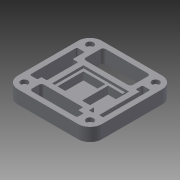
# Autodesk Inventor part: 16 pin holder
Saved by Autodesk Inventor 2015 (Build 190159000, 159)
## iProperties
Created: 2014-12-11
Part Number: 16 pin holder
Material: Generic
Document SubType Name: Modeling
Designer: Purple
Density: 1 g/cm^3
Appearance: Default
Author: Purple
Autodesk Inventor part; units mm, degrees
ref_plane "YZ Plane" through (0, 0, 0) normal (1, 0, 0) x (0, 1, 0)
ref_plane "XZ Plane" through (0, 0, 0) normal (0, 1, 0) x (-1, 0, 0)
sketch "Sketch1" plane through (0, 0, 0) normal (0, 1, 0) x (-1, 0, 0)
  line L0 (30, 30) -> (-30, 30)
  line L1 (-30, 30) -> (-30, -30)
  line L2 (-30, -30) -> (30, -30)
  line L3 (30, -30) -> (30, 30)
  line L4 (30, 30) -> (-30, -30) construction
  line L5 (-30, 30) -> (30, -30) construction
  point P0 (0, 0)
  dimension "d0" = 60
  dimension "d1" = 60
  constraints: 12 end point, 2 midpoint, 2 parallel, 1 horizontal, 1 perpendicular
  measures "d0" distance of L2.end L1.end
  measures "d1" distance of L0.end L1.end
extrude "Extrusion1" add sketch "Sketch1" along normal blind 10
fillet "Fillet1" radius 7 4 edges at (30, 5, 30) (30, 5, -30) (-30, 5, 30) (-30, 5, -30)
sketch "Sketch2" plane through (0, 10, 0) normal (0, 1, 0) x (1, 0, 0)
  line L0 (-30, 30) -> (30, 30)
  line L1 (30, 30) -> (30, -30)
  line L2 (30, -30) -> (-30, -30)
  line L3 (-30, -30) -> (-30, 30)
  line L4 (-30, 30) -> (30, -30) construction
  line L5 (30, 30) -> (-30, -30) construction
  line L6 (25, -25) -> (25, 25)
  line L7 (25, 25) -> (-25, 25)
  line L8 (-25, 25) -> (-25, -25)
  line L9 (-25, -25) -> (25, -25)
  circle A0 centre (25, -25) radius 2.75
  circle A1 centre (-25, -25) radius 2.75
  circle A2 centre (25, 25) radius 2.75
  circle A3 centre (-25, 25) radius 2.75
  point P0 (0, 0)
  dimension "d5" = 5
  dimension "d6" = 5.5
  dimension "d7" = 5.5
  dimension "d8" = 5.5
  dimension "d9" = 5.5
  constraints: 20 end point, 4 centre point, 4 coincident, 4 parallel, 2 midpoint, 2 perpendicular, 1 horizontal, 3 other
  measures "d5" distance between parallel lines of L1 L6
  measures "d6" diameter of A0
  measures "d7" diameter of A1
  measures "d8" diameter of A2
  measures "d9" diameter of A3
extrude "Extrusion2" cut sketch "Sketch2" against normal blind 3 contours L9 A0 L6 | L6 A0 L9 | A2 L7 L6 | L6 L7 A2 | A1 L8 L9 | L9 L8 A1 | A3 L8 L7 | L7 L8 A3
sketch "Sketch7" plane through (0, 10, 0) normal (0, 1, 0) x (1, 0, 0)
  line L0 (-23, 30) -> (23, 30)
  line L1 (30, 23) -> (30, -23)
  line L2 (23, -30) -> (-23, -30)
  line L3 (-30, -23) -> (-30, 23)
  line L4 (-30, 30) -> (30, -30) construction
  line L5 (30, 30) -> (-30, -30) construction
  arc A0 (-23, 30) -> (-30, 23) centre (-23, 23) ccw
  arc A1 (-30, -23) -> (-23, -30) centre (-23, -23) ccw
  arc A2 (23, -30) -> (30, -23) centre (23, -23) ccw
  arc A3 (30, 23) -> (23, 30) centre (23, 23) ccw
  line L6 (23, 32) -> (-23, 32)
  arc A4 (-23, 32) -> (-32, 23) centre (-23, 23) ccw
  line L7 (-32, 23) -> (-32, -23)
  arc A5 (-32, -23) -> (-23, -32) centre (-23, -23) ccw
  line L8 (-23, -32) -> (23, -32)
  arc A6 (23, -32) -> (32, -23) centre (23, -23) ccw
  line L9 (32, -23) -> (32, 23)
  arc A7 (32, 23) -> (23, 32) centre (23, 23) ccw
  point P0 (0, 0)
  dimension "d47" = 7
  dimension "d48" = 2
  constraints: 20 end point, 16 point on circle, 8 centre point, 8 point on line, 8 tangent, 4 parallel, 3 equal radius, 2 midpoint, 2 perpendicular, 1 horizontal, 7 other
  measures "d47" radius of A0
  measures "d48" distance between parallel lines of L0 L6
extrude "Extrusion6" add sketch "Sketch7" against normal blind 10
sketch "Sketch23" plane through (0, 10, 0) normal (0, 1, 0) x (1, 0, 0)
  line L0 (-25, 25) -> (25, 25)
  line L1 (25, 25) -> (25, -25)
  line L2 (25, -25) -> (-25, -25)
  line L3 (-25, -25) -> (-25, 25)
  line L4 (-25, 25) -> (25, -25) construction
  line L5 (25, 25) -> (-25, -25) construction
  line L6 (21, -21) -> (21, 21)
  line L7 (21, 21) -> (-21, 21)
  line L8 (-21, 21) -> (-21, -21)
  line L9 (-21, -21) -> (21, -21)
  line L10 (-13.8, -15) -> (-13.8, 8.8)
  line L11 (-13.8, 8.8) -> (21, 8.8)
  line L12 (-11.8, 6.8) -> (-11.8, -15)
  line L13 (18, 8.8) -> (18, 6.8)
  line L14 (-13.8, -15) -> (18, -15)
  line L15 (7, 3.1073) -> (7, -15)
  line L16 (7, 3.1073) -> (7, 6.8)
  line L17 (5, -15) -> (5, 3.1073)
  line L18 (5, 3.1073) -> (5, 6.8)
  line L19 (5, 6.8) -> (-11.8, 6.8)
  line L20 (18, -15) -> (18, -18.6)
  line L21 (18, -18.6) -> (21, -18.6)
  line L22 (18, 6.8) -> (7, 6.8)
  point P0 (0, 0)
  point P1 (21, -15)
  dimension "d215" = 50
  dimension "d216" = 50
  dimension "d217" = 4
  dimension "d218" = 6
  dimension "d220" = 34.8
  dimension "d221" = 23.8
  dimension "d224" = 3
  dimension "d225" = 14
  dimension "d226" = 2
  dimension "d227" = 3
  dimension "d228" = 3.6
  constraints: 46 end point, 7 point on line, 6 perpendicular, 5 parallel, 2 horizontal, 2 midpoint, 2 vertical, 3 other
  measures "d215" distance of L1.end L2.end
  measures "d216" distance of L0.end L1.end
  measures "d217" distance between parallel lines of L1 L6
  measures "d218" distance of point (21, -15) L6.start
  measures "d220" distance of point (21, -15) L10.start
  measures "d221" distance of L11.end point (21, -15)
  measures "d224" distance of L11.end L13.start
  measures "d225" distance from line of L15.start L6
  measures "d226" distance between parallel lines of L15 L17
  measures "d227" distance of L14.end point (21, -15)
  measures "d228" distance of L14.end L20.end
extrude "Extrusion21" cut sketch "Sketch23" against normal blind 2 contours L13 L22 L16 L15 L14 L17 L18 L19 L12 L10 L11
sketch "Sketch24" plane through (0, 10, 0) normal (0, 1, 0) x (1, 0, 0)
  line L0 (-11.8, 6.8) -> (5, 6.8)
  line L1 (5, 6.8) -> (5, -15)
  line L2 (5, -15) -> (-11.8, -15)
  line L3 (-11.8, -15) -> (-11.8, 6.8)
  point P0 (0, 0)
  constraints: 8 end point, 2 parallel, 1 horizontal, 1 perpendicular
extrude "Extrusion22" cut sketch "Sketch24" against normal blind 8
sketch "Sketch25" plane through (0, 10, 0) normal (0, 1, 0) x (1, 0, 0)
  line L0 (7, 6.8) -> (18, 6.8)
  line L1 (18, 6.8) -> (18, 8.8)
  line L2 (18, 8.8) -> (21, 8.8)
  line L3 (7, 6.8) -> (7, -15)
  line L4 (21, 8.8) -> (21, -15)
  line L5 (7, -15) -> (18, -15)
  line L6 (18, -15) -> (18, -18.8)
  line L7 (18, -18.8) -> (21, -18.8)
  line L8 (21, -18.8) -> (21, -15)
  point P0 (0, 0)
  point P1 (21, -17.8036)
  dimension "d233" = 3
  dimension "d234" = 3
  dimension "d235" = 3.8
  constraints: 18 end point, 3 horizontal, 3 perpendicular, 3 vertical
  measures "d233" distance of L2.end L1.end
  measures "d234" distance of L5.end L4.end
  measures "d235" distance of L5.end L6.end
extrude "Extrusion23" cut sketch "Sketch25" against normal blind 8
sketch "Sketch26" plane through (0, 10, 0) normal (0, 1, 0) x (1, 0, 0)
  line L0 (23, 32) -> (-23, 32) projected
  line L1 (-32, 23) -> (-32, -23) projected
  line L2 (32, -23) -> (32, 23) projected
  line L3 (-13.8, 8.8) -> (21, 8.8) projected
  line L4 (-18, 28) -> (-18, 12.8)
  line L5 (-18, 12.8) -> (18, 12.8)
  line L6 (18, 12.8) -> (18, 28)
  line L7 (18, 28) -> (-18, 28)
  line L8 (-23, -32) -> (23, -32) projected
  line L9 (21, 8.8) -> (21, -18.8) projected
  line L10 (28, 18) -> (28, -18)
  line L11 (28, -18) -> (25, -18)
  line L12 (25, -18) -> (25, 8.8)
  line L13 (25, 8.8) -> (25, 12.8)
  line L14 (25, 12.8) -> (22, 12.8)
  line L15 (22, 12.8) -> (22, 18)
  line L16 (22, 18) -> (28, 18)
  line L17 (21, -18.8) -> (18, -18.8) projected
  line L18 (18, -15) -> (-13.8, -15) projected
  line L19 (18, -28) -> (-18, -28)
  line L20 (-18, -28) -> (-18, -19)
  line L21 (-18, -19) -> (13.8369, -19)
  line L22 (13.8369, -19) -> (13.8369, -22.8)
  line L23 (13.8369, -22.8) -> (18, -22.8)
  line L24 (18, -22.8) -> (18, -28)
  line L25 (-13.8, -15) -> (-13.8, 8.8) projected
  line L26 (-28, 18) -> (-22, 18)
  line L27 (-22, 18) -> (-22, 8.8)
  line L28 (-22, 8.8) -> (-17.8, 8.8)
  line L29 (-17.8, 8.8) -> (-17.8, -15)
  line L30 (-17.8, -15) -> (-22, -15)
  line L31 (-22, -15) -> (-22, -18)
  line L32 (-22, -18) -> (-28, -18)
  line L33 (-28, -18) -> (-28, 18)
  point P0 (0, 0)
  dimension "d238" = 4
  dimension "d239" = 4
  dimension "d240" = 14
  dimension "d241" = 14
  dimension "d242" = 4
  dimension "d243" = 4
  dimension "d244" = 14
  dimension "d245" = 4
  dimension "d246" = 14
  dimension "d247" = 4
  dimension "d248" = 4
  dimension "d249" = 4
  dimension "d250" = 4
  dimension "d251" = 14
  dimension "d252" = 14
  dimension "d253" = 4
  dimension "d254" = 4
  dimension "d255" = 4
  dimension "d256" = 14
  dimension "d257" = 4
  dimension "d258" = 14
  dimension "d259" = 4
  dimension "d260" = 4
  constraints: 50 end point, 16 perpendicular, 2 horizontal, 1 parallel, 1 point on line, 1 vertical
  measures "d238" distance from line of L4.start L0
  measures "d239" distance from line of L6.end L0
  measures "d240" distance from line of L1 L4.start
  measures "d241" distance from line of L2 L6.end
  measures "d242" distance from line of L4.end L3
  measures "d243" distance from line of L2 L10.start
  measures "d244" distance from line of L0 L10.start
  measures "d245" distance from line of L2 L10.end
  measures "d246" distance from line of L8 L10.end
  measures "d247" distance from line of L15.end L6
  measures "d248" distance from line of L9 L12.end
  measures "d249" distance from line of L8 L19.start
  measures "d250" distance from line of L8 L19.end
  measures "d251" distance from line of L2 L19.start
  measures "d252" distance from line of L1 L19.end
  measures "d253" distance from line of L23.end L17
  measures "d254" distance from line of L21.end L18
  measures "d255" distance from line of L26.start L1
  measures "d256" distance from line of L26.start L0
  measures "d257" distance from line of L1 L32.end
  measures "d258" distance from line of L8 L32.end
  measures "d259" distance from line of L31.end L20
  measures "d260" distance from line of L29.end L25
extrude "Extrusion24" cut sketch "Sketch26" against normal through all
fillet "Fillet7" radius 0.5 13 edges at (-22, 5, -18) (-22, 5, -8.8) (-17.8, 5, -8.8) (-22, 5, 15) (-17.8, 5, 15) (-22, 5, 18) (22, 5, -12.8) (25, 5, -12.8) (28, 5, 18) (25, 5, 18) (13.8369, 5, 19) (13.8369, 5, 22.8) (18, 5, 22.8)
fillet "Fillet7" radius 1 5 edges at (22, 5, -18) (28, 5, -18) (-28, 5, -18) (-28, 5, 18) (18, 5, 28)
fillet "Fillet7" radius 2 6 edges at (-18, 5, -28) (18, 5, -28) (18, 5, -12.8) (-18, 5, -12.8) (-18, 5, 19) (-18, 5, 28)
ref_plane "Work Plane6" through (0, 5, 0) normal (0, 1, 0) x (1, 0, 0)
mirror "Mirror6" about plane through (0, 5, 0) normal (0, 1, 0) of "Extrusion2"
body "Solid1"
